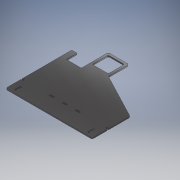
# Autodesk Inventor part: INTERNAL SIDE PLATE
Saved by Autodesk Inventor 2018 (Build 220112000, 112)
## iProperties
Created: 2018-10-15
Part Number: INTERNAL SIDE PLATE
Material: Acero, carbono
Document SubType Name: Modeling
Designer: Toshiba
Density: 7.85 g/cm^3
Appearance: Mecanizado 02
Author: Toshiba
Autodesk Inventor part; units mm, degrees
ref_plane "YZ Plane" through (0, 0, 0) normal (1, 0, 0) x (0, 1, 0)
ref_plane "XZ Plane" through (0, 0, 0) normal (0, 1, 0) x (-1, 0, 0)
ref_plane "XY Plane" through (0, 0, 0) normal (0, 0, 1) x (1, 0, 0)
sketch "Boceto1" plane through (0, 0, 0) normal (0, 0, 1) x (1, 0, 0)
  line L0 (200, -200) -> (-200, -200)
  line L1 (-200, -200) -> (-200, 105)
  line L2 (-105, 105) -> (-105, 200)
  line L3 (-105, 200) -> (-10, 200)
  line L4 (-10, 200) -> (-10, 105)
  line L5 (200, -200) -> (200, -5)
  line L6 (200, -5) -> (-10, 105)
  line L7 (-20, 115) -> (-95, 115)
  line L8 (-95, 115) -> (-95, 190)
  line L9 (-95, 190) -> (-20, 190)
  line L10 (-20, 190) -> (-20, 115)
  line L11 (-20, 115) -> (-95, 190) construction
  line L12 (-95, 115) -> (-20, 190) construction
  line L13 (-200, 105) -> (-200, 125)
  line L14 (-200, 125) -> (-175, 125)
  line L15 (-175, 125) -> (-175, 75)
  line L16 (-175, 75) -> (-105, 75)
  line L17 (-105, 75) -> (-105, 105)
  point P0 (0, 0)
  point P1 (-57.5, 152.5)
  dimension "d0" = 305
  dimension "d1" = 95
  dimension "d2" = 95
  dimension "d3" = 195
  dimension "d4" = 400
  dimension "d7" = 75
  dimension "d8" = 75
  dimension "d9" = 20
  dimension "d10" = 25
  dimension "d11" = 50
  constraints: 36 end point, 7 perpendicular, 5 vertical, 3 horizontal, 2 midpoint, 2 parallel
  measures "d0" distance of L0.end L1.end
  measures "d1" distance of L1.end L2.start
  measures "d2" distance of L2.end L3.end
  measures "d3" distance of L0.start L5.end
  measures "d4" distance of L0.start L0.end
  measures "d7" distance of L8.end L9.end
  measures "d8" distance of L7.end L8.end
  measures "d9" distance of L1.end L13.end
  measures "d10" distance of L13.end L14.end
  measures "d11" distance of L14.end L15.end
extrude "Extrusión1" add sketch "Boceto1" along normal blind 6
fillet "Empalme1" radius 2 3 edges at (-175, 125, 3) (-175, 75, 3) (-105, 75, 3)
fillet "Empalme2" radius 6 11 edges at (-200, 125, 3) (-105, 200, 3) (-10, 200, 3) (-10, 105, 3) (-95, 115, 3) (-95, 190, 3) (-20, 190, 3) (-20, 115, 3) (200, -5, 3) (200, -200, 3) (-200, -200, 3)
sketch "Boceto2" plane through (0, 0, 6) normal (0, 0, 1) x (1, 0, 0)
  line L0 (10, -110) -> (-10, -110)
  line L1 (-10, -110) -> (-10, -104)
  line L2 (-10, -104) -> (10, -104)
  line L3 (10, -104) -> (10, -110)
  line L4 (10, -110) -> (-10, -104) construction
  line L5 (-10, -110) -> (10, -104) construction
  line L6 (-50, -110) -> (-70, -110)
  line L7 (-70, -110) -> (-70, -104)
  line L8 (-70, -104) -> (-50, -104)
  line L9 (-50, -104) -> (-50, -110)
  line L10 (-50, -110) -> (-70, -104) construction
  line L11 (-70, -110) -> (-50, -104) construction
  line L12 (70, -110) -> (50, -110)
  line L13 (50, -110) -> (50, -104)
  line L14 (50, -104) -> (70, -104)
  line L15 (70, -104) -> (70, -110)
  line L16 (70, -110) -> (50, -104) construction
  line L17 (50, -110) -> (70, -104) construction
  circle A0 centre (-170, -107) radius 4
  line L18 (-190, -110) -> (-210, -110)
  line L19 (-210, -110) -> (-210, -104)
  line L20 (-210, -104) -> (-190, -104)
  line L21 (-190, -104) -> (-190, -110)
  line L22 (-200, -149) -> (-200, 99)
  line L23 (-190, -110) -> (-210, -104) construction
  line L24 (-210, -110) -> (-190, -104) construction
  line L25 (0, 0) -> (0, -107)
  line L26 (210, -104) -> (190, -104)
  line L27 (190, -110) -> (210, -110)
  line L28 (190, -104) -> (190, -110)
  line L29 (210, -110) -> (210, -104)
  point P0 (-60, -107)
  point P1 (60, -107)
  point P2 (-200, -107)
  dimension "d16" = 20
  dimension "d17" = 6
  dimension "d18" = 20
  dimension "d19" = 60
  dimension "d20" = 20
  dimension "d21" = 60
  dimension "d22" = 8
  dimension "d23" = 20
  dimension "d24" = 6
  dimension "d25" = 110
  dimension "d27" = 6
  dimension "d28" = 6
  dimension "d29" = 107
  constraints: 60 end point, 8 midpoint, 8 parallel, 5 perpendicular, 4 horizontal, 4 symmetric about line, 1 centre point, 1 point on line
  measures "d16" distance of L1.end L3.start
  measures "d17" distance of L1.start L1.end
  measures "d18" distance of L7.end L8.end
  measures "d19" distance of point (-60, -107) L25.end
  measures "d20" distance of L13.end L14.end
  measures "d21" distance of point (60, -107) L25.end
  measures "d22" diameter of A0
  measures "d23" distance of L20.start L21.start
  measures "d24" distance of L18.end L20.start
  measures "d25" distance of point (-60, -107) A0.centre
  measures "d27" distance of L8.end L6.start
  measures "d28" distance of L14.end L12.start
  measures "d29" distance of L25.end L25.start
extrude "Extrusión2" cut sketch "Boceto2" against normal through all contours L0 L1 L2 L3 | L6 L7 L8 L9 | L12 L13 L14 L15 | L18 L22 L20 L21 | L18 L19 L20 L22 | L29 L27 L28 L26
sketch "Boceto3" plane through (0, 0, 6) normal (0, 0, 1) x (1, 0, 0)
  line L0 (-194, -200) -> (194, -200) projected
  line L1 (0, -200) -> (0, -130)
  line L2 (0, -130) -> (-200, -130)
  line L3 (-200, -110) -> (-200, -194) projected
  line L4 (-200, -130) -> (-200, -120)
  line L5 (-200, -120) -> (200, -120)
  line L6 (200, -110) -> (200, -194) projected
  line L7 (0, -130) -> (200, -130)
  line L8 (200, -120) -> (200, -130)
  line L9 (10, -110) -> (-10, -110)
  line L10 (-10, -110) -> (-10, -104)
  line L11 (-10, -104) -> (10, -104)
  line L12 (10, -104) -> (10, -110)
  line L13 (10, -110) -> (-10, -104) construction
  line L14 (-10, -110) -> (10, -104) construction
  line L15 (-50, -110) -> (-70, -110)
  line L16 (-70, -110) -> (-70, -104)
  line L17 (-70, -104) -> (-50, -104)
  line L18 (-50, -104) -> (-50, -110)
  line L19 (-50, -110) -> (-70, -104) construction
  line L20 (-70, -110) -> (-50, -104) construction
  line L21 (70, -110) -> (50, -110)
  line L22 (50, -110) -> (50, -104)
  line L23 (50, -104) -> (70, -104)
  line L24 (70, -104) -> (70, -110)
  line L25 (70, -110) -> (50, -104) construction
  line L26 (50, -110) -> (70, -104) construction
  circle A0 centre (-170, -107) radius 4
  line L27 (-190, -110) -> (-210, -110)
  line L28 (-210, -110) -> (-210, -104)
  line L29 (-210, -104) -> (-190, -104)
  line L30 (-190, -104) -> (-190, -110)
  line L31 (-200, -149) -> (-200, 99)
  line L32 (-190, -110) -> (-210, -104) construction
  line L33 (-210, -110) -> (-190, -104) construction
  circle A1 centre (-80, -95) radius 3
  circle A2 centre (-80, -51) radius 3
  circle A3 centre (-170, -80) radius 3
  circle A4 centre (-170, -60) radius 3
  line L34 (0, 0) -> (0, -107)
  circle A5 centre (170, -107) radius 4
  line L35 (210, -104) -> (190, -104)
  line L36 (190, -110) -> (210, -110)
  line L37 (190, -104) -> (190, -110)
  line L38 (210, -110) -> (210, -104)
  circle A6 centre (80, -95) radius 3
  circle A7 centre (80, -51) radius 3
  circle A8 centre (170, -107) radius 13
  circle A9 centre (-170, -107) radius 13
  circle A10 centre (-170, -143) radius 13
  circle A11 centre (-170, -143) radius 4
  circle A12 centre (-170, -165) radius 4
  line L39 (-174, -143) -> (-174, -165)
  line L40 (-166, -165) -> (-166, -143)
  circle A13 centre (170, -143) radius 13
  circle A14 centre (170, -143) radius 4
  circle A15 centre (170, -165) radius 4
  line L41 (174, -143) -> (174, -165)
  line L42 (166, -165) -> (166, -143)
  point P0 (-60, -107)
  point P1 (60, -107)
  point P2 (-200, -107)
  dimension "d33" = 70
  dimension "d34" = 10
  dimension "d35" = 20
  dimension "d36" = 6
  dimension "d38" = 20
  dimension "d39" = 60
  dimension "d40" = 20
  dimension "d41" = 60
  dimension "d42" = 8
  dimension "d43" = 20
  dimension "d44" = 6
  dimension "d45" = 110
  dimension "d46" = 6
  dimension "d47" = 20
  dimension "d48" = 12
  dimension "d49" = 6
  dimension "d50" = 44
  dimension "d51" = 6
  dimension "d52" = 6
  dimension "d54" = 6
  dimension "d55" = 6
  dimension "d56" = 26
  dimension "d57" = 8
  dimension "d58" = 8
  constraints: 80 end point, 16 centre point, 14 symmetric about line, 9 midpoint, 9 parallel, 8 point on circle, 7 perpendicular, 6 point on line, 4 coincident, 4 horizontal, 3 tangent, 2 vertical, 1 collinear, 6 other
  measures "d33" distance of L1.start L1.end
  measures "d34" distance of L2.end L4.end
  measures "d35" distance of L10.end L11.end
  measures "d36" distance of L9.end L10.end
  measures "d38" distance of L16.end L17.end
  measures "d39" distance of point (-60, -107) L34.end
  measures "d40" distance of L22.end L23.end
  measures "d41" distance of point (60, -107) L34.end
  measures "d42" diameter of A0
  measures "d43" distance of L28.end L29.end
  measures "d44" distance of L27.end L28.end
  measures "d45" distance of point (-60, -107) A0.centre
  measures "d46" diameter of A1
  measures "d47" horizontal distance of A1.centre point (-60, -107)
  measures "d48" vertical distance of point (-60, -107) A1.centre
  measures "d49" diameter of A2
  measures "d50" distance of A1.centre A2.centre
  measures "d51" diameter of A3
  measures "d52" diameter of A4
  measures "d54" distance of L17.end L15.start
  measures "d55" distance of L23.end L21.start
  measures "d56" diameter of A10
  measures "d57" diameter of A11
  measures "d58" diameter of A12
extrude "Extrusión3" cut sketch "Boceto3" against normal through all contours L39 A11 L40 A10 | A10 L40 A12 L39 | L42 A14 L41 A13 | A13 L41 A15 L42 | A11 | A12 | A15 | A14 picked at (-169.8393, -152.9432) picked at (170.1607, -152.9432)
sketch "Boceto5" plane through (0, 0, 6) normal (0, 0, 1) x (1, 0, 0)
  line L0 (-194, -200) -> (194, -200) projected
  line L1 (0, -200) -> (200, -200)
  line L2 (200, -200) -> (200, -180)
  line L3 (200, -194) -> (200, -110) projected
  line L4 (200, -180) -> (-200, -180)
  line L5 (-200, -110) -> (-200, -194) projected
  line L6 (-200, -200) -> (-200, -180)
  line L7 (-200, -200) -> (0, -200)
  point P0 (0, 0)
  dimension "d61" = 20
  constraints: 10 end point, 3 perpendicular, 3 point on line, 1 horizontal, 1 midpoint
  measures "d61" distance of L1.end L2.end
extrude "Extrusión4" cut sketch "Boceto5" against normal through all
fillet "Empalme3" radius 6 2 edges at (-200, -180, 3) (200, -180, 3)
